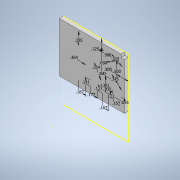
# Autodesk Inventor part: magnet_hall_testing
Saved by Autodesk Inventor 2021 (Build 250183000, 183)
## iProperties
Created: 2021-02-24
Part Number: magnet_hall_testing
Material: Generic
Document SubType Name: Modeling
Designer: Patrick
Density: 1 g/cm^3
Appearance: Default
Author: Patrick
Autodesk Inventor part; units mm, degrees
ref_plane "YZ Plane" through (0, 0, 0) normal (1, 0, 0) x (0, 1, 0)
ref_plane "XZ Plane" through (0, 0, 0) normal (0, 1, 0) x (-1, 0, 0)
ref_plane "XY Plane" through (0, 0, 0) normal (0, 0, 1) x (1, 0, 0)
sketch "Sketch2" plane through (0, 0, 0) normal (0, 0, 1) x (1, 0, 0)
  line L0 (7.62, 67.0577) -> (50.8, 67.0577)
  line L1 (50.8, 67.0577) -> (50.8, 16.2577)
  line L2 (50.8, 16.2577) -> (7.62, 16.2577)
  line L3 (7.62, 16.2577) -> (7.62, 67.0577)
  point P0 (0, 0)
  dimension "d45" = 43.18
  dimension "d46" = 50.8
  constraints: 8 end point, 2 parallel, 1 horizontal, 1 perpendicular
  measures "d45" distance of L1.end L2.end
  measures "d46" distance of L0.end L1.end
extrude "Extrusion1" add sketch "Sketch2" along normal blind 2.54
sketch "Sketch3" plane through (0, 0, 0) normal (0, 0, -1) x (-1, 0, 0)
  circle A0 centre (-43.18, 59.4377) radius 4.0005
  line L0 (-50.8, 16.2577) -> (-50.8, 67.0577) projected
  line L1 (-50.8, 67.0577) -> (-7.62, 67.0577) projected
  circle A1 centre (-43.18, 59.4377) radius 5.2705
  line L2 (-7.62, 67.0577) -> (-7.62, 16.2577) projected
  line L3 (-7.62, 16.2577) -> (-50.8, 16.2577) projected
  circle A2 centre (-43.18, 46.7377) radius 5.2705
  circle A3 centre (-30.48, 59.4377) radius 5.2705
  circle A4 centre (-30.48, 46.7377) radius 5.2705
  circle A5 centre (-17.78, 59.4377) radius 5.2705
  circle A6 centre (-17.78, 46.7377) radius 5.2705
  line L4 (-45.1739, 39.1092) -> (-41.1861, 39.1092)
  line L5 (-41.1861, 39.1092) -> (-41.1861, 36.0358)
  line L6 (-41.1861, 36.0358) -> (-45.1739, 36.0358)
  line L7 (-45.1739, 36.0358) -> (-45.1739, 39.1092)
  line L8 (-45.1739, 39.1092) -> (-41.1861, 36.0358) construction
  line L9 (-41.1861, 39.1092) -> (-45.1739, 36.0358) construction
  line L10 (-45.9813, 35.4135) -> (-40.3787, 35.4135)
  line L11 (-40.3787, 35.4135) -> (-40.3787, 39.7315)
  line L12 (-40.3787, 39.7315) -> (-45.9813, 39.7315)
  line L13 (-45.9813, 39.7315) -> (-45.9813, 35.4135)
  line L14 (-45.9813, 35.4135) -> (-40.3787, 39.7315) construction
  line L15 (-40.3787, 35.4135) -> (-45.9813, 39.7315) construction
  circle A7 centre (-30.48, 59.4377) radius 4.1255
  circle A8 centre (-17.78, 59.4377) radius 4.2505
  circle A9 centre (-43.18, 46.7377) radius 4.3755
  circle A10 centre (-30.48, 46.7377) radius 4.5005
  circle A11 centre (-17.78, 46.7377) radius 4.6255
  line L16 (-32.7587, 39.7315) -> (-38.3613, 39.7315)
  line L17 (-38.3613, 39.7315) -> (-38.3613, 35.4135)
  line L18 (-38.3613, 35.4135) -> (-32.7587, 35.4135)
  line L19 (-32.7587, 35.4135) -> (-32.7587, 39.7315)
  line L20 (-25.1387, 39.7315) -> (-30.7413, 39.7315)
  line L21 (-30.7413, 39.7315) -> (-30.7413, 35.4135)
  line L22 (-30.7413, 35.4135) -> (-25.1387, 35.4135)
  line L23 (-25.1387, 35.4135) -> (-25.1387, 39.7315)
  line L24 (-17.5187, 39.7315) -> (-23.1213, 39.7315)
  line L25 (-23.1213, 39.7315) -> (-23.1213, 35.4135)
  line L26 (-23.1213, 35.4135) -> (-17.5187, 35.4135)
  line L27 (-17.5187, 35.4135) -> (-17.5187, 39.7315)
  line L28 (-9.8987, 39.7315) -> (-15.5013, 39.7315)
  line L29 (-15.5013, 39.7315) -> (-15.5013, 35.4135)
  line L30 (-15.5013, 35.4135) -> (-9.8987, 35.4135)
  line L31 (-9.8987, 35.4135) -> (-9.8987, 39.7315)
  line L32 (-37.6789, 35.9108) -> (-33.4411, 35.9108)
  line L33 (-33.4411, 35.9108) -> (-33.4411, 39.2342)
  line L34 (-33.4411, 39.2342) -> (-37.6789, 39.2342)
  line L35 (-37.6789, 39.2342) -> (-37.6789, 35.9108)
  line L36 (-37.6789, 35.9108) -> (-33.4411, 39.2342) construction
  line L37 (-33.4411, 35.9108) -> (-37.6789, 39.2342) construction
  line L38 (-30.1839, 35.7858) -> (-25.6961, 35.7858)
  line L39 (-25.6961, 35.7858) -> (-25.6961, 39.3592)
  line L40 (-25.6961, 39.3592) -> (-30.1839, 39.3592)
  line L41 (-30.1839, 39.3592) -> (-30.1839, 35.7858)
  line L42 (-30.1839, 35.7858) -> (-25.6961, 39.3592) construction
  line L43 (-25.6961, 35.7858) -> (-30.1839, 39.3592) construction
  line L44 (-22.6889, 35.6608) -> (-17.9511, 35.6608)
  line L45 (-17.9511, 35.6608) -> (-17.9511, 39.4842)
  line L46 (-17.9511, 39.4842) -> (-22.6889, 39.4842)
  line L47 (-22.6889, 39.4842) -> (-22.6889, 35.6608)
  line L48 (-22.6889, 35.6608) -> (-17.9511, 39.4842) construction
  line L49 (-17.9511, 35.6608) -> (-22.6889, 39.4842) construction
  line L50 (-45.1739, 35.3552) -> (-41.1861, 35.3552)
  line L51 (-41.1861, 35.3552) -> (-41.1861, 36.7164)
  line L52 (-41.1861, 36.7164) -> (-45.1739, 36.7164)
  line L53 (-45.1739, 36.7164) -> (-45.1739, 35.3552)
  line L54 (-45.1739, 35.3552) -> (-41.1861, 36.7164) construction
  line L55 (-41.1861, 35.3552) -> (-45.1739, 36.7164) construction
  point P0 (0, 0)
  point P1 (-43.18, 37.5725)
  point P2 (-43.18, 37.5725)
  point P3 (-35.56, 37.5725)
  point P4 (-27.94, 37.5725)
  point P5 (-20.32, 37.5725)
  point P6 (-12.7, 37.5725)
  point P7 (-43.18, 36.0358)
  dimension "d49" = 7.62
  dimension "d50" = 7.62
  dimension "d51" = 1.27
  dimension "d56" = 12.7
  dimension "d59" = 12.7
  dimension "d64" = 3.9878
  dimension "d65" = 3.0734
  dimension "d66" = 9.1652
  dimension "d67" = 2.159
  dimension "d77" = 8.001
  dimension "d78" = 8.251
  dimension "d80" = 8.501
  dimension "d81" = 8.751
  dimension "d82" = 9.001
  dimension "d83" = 9.251
  dimension "d90" = 7.62
  dimension "d95" = 4.2378
  dimension "d96" = 4.4878
  dimension "d97" = 4.7378
  dimension "d98" = 3.3234
  dimension "d99" = 3.5734
  constraints: 104 end point, 14 midpoint, 12 centre point, 12 parallel, 8 horizontal, 6 coincident, 6 perpendicular, 2 point on line, 1 vertical, 1 vertical alignment, 46 other
  measures "d49" distance from line of A0.centre L0
  measures "d50" distance from line of L1 A0.centre
  measures "d51" radial gap between concentric circles of A1 A0
  measures "d56" distance of A1.centre A2.centre
  measures "d59" distance of A1.centre A3.centre
  measures "d64" distance of L5.end L6.end
  measures "d65" distance of L5.end L4.end
  measures "d66" distance of A2.centre point (-43.18, 37.573)
  measures "d67" vertical distance of L12.end point (-43.18, 37.573)
  measures "d77" diameter of A0
  measures "d78" diameter of A7
  measures "d80" diameter of A8
  measures "d81" diameter of A9
  measures "d82" diameter of A10
  measures "d83" diameter of A11
  measures "d90" distance of L11.end L16.start
  measures "d95" distance between parallel lines of L33 L35
  measures "d96" distance between parallel lines of L39 L41
  measures "d97" distance between parallel lines of L45 L47
  measures "d98" distance between parallel lines of L32 L34
  measures "d99" distance between parallel lines of L38 L40
sketch "Sketch4" plane through (0, 0, 0) normal (0, 0, -1) x (-1, 0, 0)
  line L0 (-50.8, 67.0577) -> (-7.62, 67.0577) projected
  line L1 (-50.8, 16.2577) -> (-50.8, 67.0577) projected
  line L2 (-50.8, 67.0577) -> (-48.5295, 67.0577)
  line L3 (-48.5295, 67.0577) -> (-48.5295, 65.0024)
  line L4 (-48.5295, 65.0024) -> (-50.8, 65.0024)
  line L5 (-50.8, 65.0024) -> (-50.8, 67.0577)
  point P0 (0, 0)
  constraints: 8 end point, 2 parallel, 1 horizontal, 1 perpendicular
extrude "Extrusion3" cut sketch "Sketch4" against normal blind 2.54
sketch "Sketch5" plane through (0, 0, 0) normal (0, 0, -1) x (-1, 0, 0)
  line L0 (-45.1739, 39.1092) -> (-41.1861, 39.1092)
  line L1 (-41.1861, 39.1092) -> (-41.1861, 36.0358)
  line L2 (-41.1861, 36.0358) -> (-45.1739, 36.0358)
  line L3 (-45.1739, 36.0358) -> (-45.1739, 39.1092)
  line L4 (-45.1739, 39.1092) -> (-41.1861, 36.0358) construction
  line L5 (-41.1861, 39.1092) -> (-45.1739, 36.0358) construction
  line L6 (-45.9813, 35.4135) -> (-40.3787, 35.4135)
  line L7 (-40.3787, 35.4135) -> (-40.3787, 39.7315)
  line L8 (-40.3787, 39.7315) -> (-45.9813, 39.7315)
  line L9 (-45.9813, 39.7315) -> (-45.9813, 35.4135)
  line L10 (-45.9813, 35.4135) -> (-40.3787, 39.7315) construction
  line L11 (-40.3787, 35.4135) -> (-45.9813, 39.7315) construction
  line L12 (-32.7587, 39.7315) -> (-38.3613, 39.7315)
  line L13 (-38.3613, 39.7315) -> (-38.3613, 35.4135)
  line L14 (-38.3613, 35.4135) -> (-32.7587, 35.4135)
  line L15 (-32.7587, 35.4135) -> (-32.7587, 39.7315)
  line L16 (-25.1387, 39.7315) -> (-30.7413, 39.7315)
  line L17 (-30.7413, 39.7315) -> (-30.7413, 35.4135)
  line L18 (-30.7413, 35.4135) -> (-25.1387, 35.4135)
  line L19 (-25.1387, 35.4135) -> (-25.1387, 39.7315)
  line L20 (-17.5187, 39.7315) -> (-23.1213, 39.7315)
  line L21 (-23.1213, 39.7315) -> (-23.1213, 35.4135)
  line L22 (-23.1213, 35.4135) -> (-17.5187, 35.4135)
  line L23 (-17.5187, 35.4135) -> (-17.5187, 39.7315)
  line L24 (-9.8987, 39.7315) -> (-15.5013, 39.7315)
  line L25 (-15.5013, 39.7315) -> (-15.5013, 35.4135)
  line L26 (-15.5013, 35.4135) -> (-9.8987, 35.4135)
  line L27 (-37.6789, 35.9108) -> (-33.4411, 35.9108)
  line L28 (-33.4411, 35.9108) -> (-33.4411, 39.2342)
  line L29 (-33.4411, 39.2342) -> (-37.6789, 39.2342)
  line L30 (-37.6789, 39.2342) -> (-37.6789, 35.9108)
  line L31 (-37.6789, 35.9108) -> (-33.4411, 39.2342) construction
  line L32 (-33.4411, 35.9108) -> (-37.6789, 39.2342) construction
  line L33 (-30.1839, 35.7858) -> (-25.6961, 35.7858)
  line L34 (-25.6961, 35.7858) -> (-25.6961, 39.3592)
  line L35 (-25.6961, 39.3592) -> (-30.1839, 39.3592)
  line L36 (-30.1839, 39.3592) -> (-30.1839, 35.7858)
  line L37 (-30.1839, 35.7858) -> (-25.6961, 39.3592) construction
  line L38 (-25.6961, 35.7858) -> (-30.1839, 39.3592) construction
  line L39 (-22.6889, 35.6608) -> (-17.9511, 35.6608)
  line L40 (-17.9511, 35.6608) -> (-17.9511, 39.4842)
  line L41 (-17.9511, 39.4842) -> (-22.6889, 39.4842)
  line L42 (-22.6889, 39.4842) -> (-22.6889, 35.6608)
  line L43 (-22.6889, 35.6608) -> (-17.9511, 39.4842) construction
  line L44 (-17.9511, 35.6608) -> (-22.6889, 39.4842) construction
  line L45 (-45.1516, 35.2931) -> (-41.1861, 36.7869) construction
  line L46 (-41.1861, 35.3552) -> (-45.1739, 36.7164) construction
  line L47 (-44.9867, 35.3552) -> (-41.3733, 35.3552)
  line L48 (-41.3733, 35.3552) -> (-41.3733, 36.7164)
  line L49 (-41.3733, 36.7164) -> (-44.9867, 36.7164)
  line L50 (-44.9867, 36.7164) -> (-44.9867, 35.3552)
  line L51 (-44.9867, 35.3552) -> (-41.3733, 36.7164) construction
  line L52 (-41.3733, 35.3552) -> (-44.9867, 36.7164) construction
  line L53 (-37.5427, 35.3747) -> (-33.5773, 35.3747)
  line L54 (-33.5773, 35.3747) -> (-33.5773, 36.447)
  line L55 (-33.5773, 36.447) -> (-37.5427, 36.447)
  line L56 (-37.5427, 36.447) -> (-37.5427, 35.3747)
  line L57 (-37.5427, 35.3747) -> (-33.5773, 36.447) construction
  line L58 (-33.5773, 35.3747) -> (-37.5427, 36.447) construction
  line L59 (-30.0124, 35.3468) -> (-25.8676, 35.3468)
  line L60 (-25.8676, 35.3468) -> (-25.8676, 36.2248)
  line L61 (-25.8676, 36.2248) -> (-30.0124, 36.2248)
  line L62 (-30.0124, 36.2248) -> (-30.0124, 35.3468)
  line L63 (-30.0124, 35.3468) -> (-25.8676, 36.2248) construction
  line L64 (-25.8676, 35.3468) -> (-30.0124, 36.2248) construction
  line L65 (-22.4558, 35.2013) -> (-18.1842, 35.2013)
  line L66 (-18.1842, 35.2013) -> (-18.1842, 36.1203)
  line L67 (-18.1842, 36.1203) -> (-22.4558, 36.1203)
  line L68 (-22.4558, 36.1203) -> (-22.4558, 35.2013)
  line L69 (-22.4558, 35.2013) -> (-18.1842, 36.1203) construction
  line L70 (-18.1842, 35.2013) -> (-22.4558, 36.1203) construction
  line L71 (-45.9813, 32.6353) -> (-41.9935, 32.6353)
  line L72 (-41.9935, 32.6353) -> (-41.9935, 29.5619)
  line L73 (-41.9935, 29.5619) -> (-45.9813, 29.5619)
  line L74 (-45.9813, 29.5619) -> (-45.9813, 32.6353)
  point P0 (0, 0)
  point P1 (-43.18, 37.5725)
  point P2 (-43.18, 37.5725)
  point P3 (-35.56, 37.5725)
  point P4 (-27.94, 37.5725)
  point P5 (-20.32, 37.5725)
  point P6 (-12.7, 37.5725)
  point P7 (-43.18, 36.0358)
  point P8 (-35.56, 35.9108)
  point P9 (-27.94, 35.7858)
  point P10 (-20.32, 35.6608)
  point P11 (-22.4558, 35.4135)
  point P12 (-22.4558, 35.6608)
  point P13 (-18.1842, 35.6608)
  point P14 (-18.1842, 35.4135)
  point P15 (-30.0124, 35.4135)
  point P16 (-30.0124, 35.7858)
  point P17 (-25.8676, 35.7858)
  point P18 (-25.8676, 35.4135)
  point P19 (-37.5427, 35.4135)
  point P20 (-37.5427, 35.9108)
  point P21 (-33.5773, 35.9108)
  point P22 (-33.5773, 35.4135)
  point P23 (-44.9867, 35.4135)
  point P24 (-44.9867, 36.0358)
  point P25 (-41.3733, 36.0358)
  point P26 (-41.3733, 35.4135)
  dimension "d102" = 3.0734
  dimension "d103" = 2.159
  dimension "d104" = 7.62
  dimension "d106" = 4.4878
  dimension "d107" = 4.7378
  dimension "d108" = 3.3234
  dimension "d109" = 3.5734
  dimension "d114" = 4.2378
  dimension "d115" = 3.0734
  dimension "d116" = 3.9878
  constraints: 150 end point, 24 midpoint, 20 parallel, 10 horizontal, 10 perpendicular, 4 point on line
  measures "d102" distance of L2.start L1.start
  measures "d103" vertical distance of L9.start point (-43.18, 37.573)
  measures "d104" distance of L10.end L15.end
  measures "d106" distance between parallel lines of L34 L36
  measures "d107" distance between parallel lines of L40 L42
  measures "d108" distance between parallel lines of L27 L29
  measures "d109" distance between parallel lines of L33 L35
  measures "d114" distance between parallel lines of L28 L30
  measures "d115" distance between parallel lines of L73 L71
  measures "d116" distance between parallel lines of L72 L74
extrude "Extrusion5" add sketch "Sketch5" along normal blind 2.54 contours L3 L2 L50 L6 L9 L8 L7 L48 L1 L0 | L15 L14 L54 L27 L28 L29 L30 L56 L13 L12 | L19 L18 L60 L33 L34 L35 L36 L62 L17 L16 | L23 L22 L66 L39 L40 L41 L42 L68 L21 L20
sketch "Sketch6" plane through (0, 0, 0) normal (0, 0, -1) x (-1, 0, 0)
  line L0 (-52.3953, 34.0161) -> (-4.7261, 34.0161)
  line L1 (-4.7261, 34.0161) -> (-4.7261, 12.2528)
  line L2 (-4.7261, 12.2528) -> (-52.3953, 12.2528)
  line L3 (-52.3953, 12.2528) -> (-52.3953, 34.0161)
  point P0 (0, 0)
  constraints: 8 end point, 2 parallel, 1 horizontal, 1 perpendicular
extrude "Extrusion6" cut sketch "Sketch6" against normal blind 2.54
body "Solid1"
